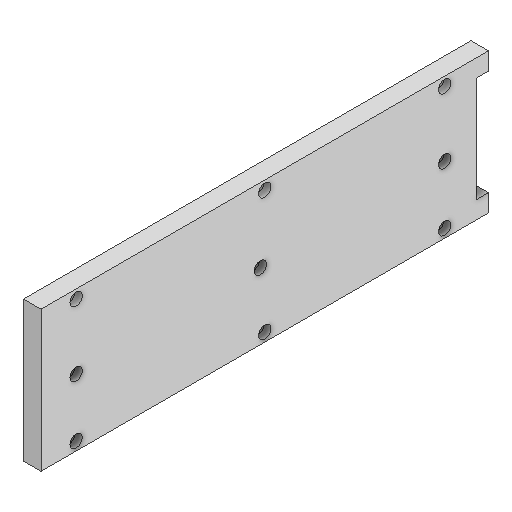
# Autodesk Inventor part: ER_Wand_1
Saved by Autodesk Inventor 2025.1 (Build 291241000, 241)
## iProperties
Created: 2025-06-25
Part Number: ER_Wand_1
Material: Generic
Document SubType Name: Modeling
Designer: Erik
Density: 1 g/cm^3
Appearance: Default
Author: Erik
Autodesk Inventor part; units mm, degrees
ref_plane "YZ Plane" through (0, 0, 0) normal (1, 0, 0) x (0, 1, 0)
ref_plane "XZ Plane" through (0, 0, 0) normal (0, 1, 0) x (-1, 0, 0)
ref_plane "XY Plane" through (0, 0, 0) normal (0, 0, 1) x (1, 0, 0)
sketch "Skizze1" plane through (0, 0, 0) normal (1, 0, 0) x (0, 1, 0)
  line L0 (-40, 127.5) -> (40, 127.5)
  line L1 (40, 127.5) -> (40, -127.5)
  line L2 (40, -127.5) -> (-40, -127.5)
  line L3 (-40, -127.5) -> (-40, 127.5)
  line L4 (-40, 127.5) -> (40, -127.5) construction
  line L5 (40, 127.5) -> (-40, -127.5) construction
  point P0 (0, 0)
  dimension "d0" = 80
  dimension "d1" = 255
  constraints: 12 end point, 2 midpoint, 2 parallel, 1 horizontal, 1 perpendicular
  measures "d0" distance of L1.end L2.end
  measures "d1" distance between parallel lines of L0 L2
extrude "Extrusion1" add sketch "Skizze1" along normal blind 10
sketch "Skizze2" plane through (10, 0, 0) normal (1, 0, 0) x (0, 0, -1)
  line L0 (-127.5, 40) -> (-127.5, -40) projected
  line L1 (127.5, -40) -> (127.5, 40) projected
  line L2 (127.5, 40) -> (-127.5, 40) projected
  line L3 (-127.5, -35) -> (127.5, -35) construction
  line L4 (-127.5, -40) -> (127.5, -40) projected
  line L5 (178.5, 0) -> (-178.5, 0) projected
  point P0 (0, 0)
  point P1 (-107.5, -2)
  point P2 (-2.5, -2)
  point P3 (102.5, -2)
  point P4 (-107.5, -35)
  point P5 (0, -35)
  point P6 (102.5, -35)
  point P7 (-107.5, 35)
  point P8 (0, 35)
  point P9 (102.5, 35)
  dimension "d4" = 20
  dimension "d5" = 25
  dimension "d6" = 105
  dimension "d7" = 42
  dimension "d8" = 42
  dimension "d9" = 42
  dimension "d27" = 5
  constraints: 4 point on line, 3 symmetric about line, 2 end point, 1 midpoint, 1 parallel
  measures "d4" distance from line of L0 point (-107.5, -2)
  measures "d5" distance from line of L1 point (102.5, -2)
  measures "d6" distance of point (-2.5, -2) point (102.5, -2)
  measures "d7" distance from line of L2 point (-107.5, -2)
  measures "d8" distance from line of point (-2.5, -2) L2
  measures "d9" distance from line of L2 point (102.5, -2)
  measures "d27" distance between parallel lines of L4 L3
hole "Bohrung1" at (10, -2, 107.5) at (10, -2, 2.5) at (10, -2, -102.5) at (10, -35, 107.5) at (10, -35, 0) at (10, -35, -102.5) at (10, 35, -102.5) at (10, 35, 0) at (10, 35, 107.5) direction (-1, 0, 0) diameter 3.242 end through all counterbore diameter 7 counterbore depth 4 thread size "M4x0.7" class "6H" standard "ISO Metric profile"
sketch "Skizze5" plane through (10, 0, 0) normal (1, 0, 0) x (0, 0, -1)
  line L0 (127.5, -40) -> (127.5, 40) projected
  line L1 (127.5, -30) -> (120.5, -30)
  line L2 (120.5, -30) -> (120.5, 30)
  line L3 (120.5, 30) -> (127.5, 30)
  line L4 (127.5, 30) -> (127.5, -30)
  line L5 (-127.5, -40) -> (127.5, -40) projected
  point P0 (0, 0)
  point P1 (124, -30)
  point P2 (124, 30)
  dimension "d28" = 7
  dimension "d29" = 60
  dimension "d30" = 10
  constraints: 8 end point, 2 midpoint, 2 parallel, 1 horizontal, 1 perpendicular, 1 point on line
  measures "d28" distance between parallel lines of L2 L0
  measures "d29" distance of point (124, -30) point (124, 30)
  measures "d30" distance from line of L5 point (124, -30)
extrude "Extrusion2" cut sketch "Skizze5" against normal blind 10
equation "\"d8\" = d7"
equation "\"d9\" = d7"
